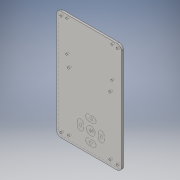
# Autodesk Inventor part: FrontCover
Saved by Autodesk Inventor 2016 (Build 200138000, 138)
## iProperties
Created: 2016-07-10
Part Number: FrontCover
Material: Generic
Document SubType Name: Modeling
Designer: jeffkub
Density: 1 g/cm^3
Appearance: Default
Author: jeffkub
Autodesk Inventor part; units mm, degrees
ref_plane "YZ Plane" through (0, 0, 0) normal (1, 0, 0) x (0, 1, 0)
ref_plane "XZ Plane" through (0, 0, 0) normal (0, 1, 0) x (-1, 0, 0)
ref_plane "XY Plane" through (0, 0, 0) normal (0, 0, 1) x (1, 0, 0)
sketch "Sketch1" plane through (0, 0, 0) normal (0, 0, 1) x (1, 0, 0)
  line L0 (30.48, -47.625) -> (-30.48, -47.625) construction
  line L1 (-34.925, -43.18) -> (-34.925, 43.18) construction
  line L2 (-30.48, 47.625) -> (30.48, 47.625) construction
  line L3 (34.925, 43.18) -> (34.925, -43.18) construction
  line L4 (34.925, -47.625) -> (-34.925, 47.625) construction
  line L5 (-34.925, -47.625) -> (34.925, 47.625) construction
  arc A0 (-30.48, 47.625) -> (-34.925, 43.18) centre (-30.48, 43.18) ccw construction
  arc A1 (34.925, 43.18) -> (30.48, 47.625) centre (30.48, 43.18) ccw construction
  arc A2 (30.48, -47.625) -> (34.925, -43.18) centre (30.48, -43.18) ccw construction
  arc A3 (-34.925, -43.18) -> (-30.48, -47.625) centre (-30.48, -43.18) ccw construction
  circle A4 centre (-30.48, 43.18) radius 1.5
  circle A5 centre (30.48, 43.18) radius 1.5
  circle A6 centre (-30.48, -43.18) radius 1.5
  circle A7 centre (30.48, -43.18) radius 1.5
  circle A8 centre (0, -22.86) radius 6.35
  line L6 (-3.175, -7.62) -> (3.175, -7.62) construction
  line L7 (-3.175, -12.065) -> (3.175, -12.065)
  line L8 (3.175, -3.175) -> (-3.175, -3.175)
  arc A9 (-3.175, -3.175) -> (-3.175, -12.065) centre (-3.175, -7.62) ccw
  arc A10 (3.175, -12.065) -> (3.175, -3.175) centre (3.175, -7.62) ccw
  line L9 (-35.3, 57.15) -> (35.3, 57.15) construction
  line L10 (35.3, 57.15) -> (35.3, 106.85) construction
  line L11 (35.3, 106.85) -> (-35.3, 106.85) construction
  line L12 (-35.3, 106.85) -> (-35.3, 57.15) construction
  circle A11 centre (-33.25, 104.75) radius 1.25
  circle A12 centre (33.25, 104.75) radius 1.25
  circle A13 centre (33.25, 59.25) radius 1.25
  circle A14 centre (-33.25, 59.25) radius 1.25
  line L13 (-41.275, 110.025) -> (41.275, 110.025)
  line L14 (47.625, 103.675) -> (47.625, -44.45)
  line L15 (41.275, -50.8) -> (-41.275, -50.8)
  line L16 (-47.625, -44.45) -> (-47.625, 103.675)
  arc A15 (-41.275, 110.025) -> (-47.625, 103.675) centre (-41.275, 103.675) ccw
  arc A16 (47.625, 103.675) -> (41.275, 110.025) centre (41.275, 103.675) ccw
  arc A17 (41.275, -50.8) -> (47.625, -44.45) centre (41.275, -44.45) ccw
  arc A18 (-47.625, -44.45) -> (-41.275, -50.8) centre (-41.275, -44.45) ccw
  circle A19 centre (-41.275, 103.675) radius 1.5
  circle A20 centre (-41.275, -44.45) radius 1.5
  circle A21 centre (41.275, -44.45) radius 1.5
  circle A22 centre (41.275, 103.675) radius 1.5
  line L17 (-0.635, -22.225) -> (-0.635, -20.32)
  line L18 (-0.635, -20.32) -> (-3.175, -22.86)
  line L19 (-3.175, -22.86) -> (-0.635, -25.4)
  line L20 (-0.635, -25.4) -> (-0.635, -23.495)
  line L21 (-0.635, -23.495) -> (3.175, -23.495)
  line L22 (3.175, -23.495) -> (3.175, -20.32)
  line L23 (3.175, -20.32) -> (1.905, -20.32)
  line L24 (1.905, -20.32) -> (1.905, -22.225)
  line L25 (1.905, -22.225) -> (-0.635, -22.225)
  line L26 (-2.54, -8.89) -> (2.54, -8.89)
  line L27 (2.54, -8.89) -> (2.54, -7.62)
  line L28 (2.54, -7.62) -> (0, -5.08)
  line L29 (0, -5.08) -> (-2.54, -7.62)
  line L30 (-2.54, -7.62) -> (-2.54, -8.89)
  arc A23 (-19.685, -26.035) -> (-10.795, -26.035) centre (-15.24, -26.035) ccw
  line L31 (-19.685, -19.685) -> (-19.685, -26.035)
  arc A24 (-10.795, -19.685) -> (-19.685, -19.685) centre (-15.24, -19.685) ccw
  line L32 (-10.795, -26.035) -> (-10.795, -19.685)
  line L33 (-13.97, -25.4) -> (-13.97, -20.32)
  line L34 (-13.97, -20.32) -> (-15.24, -20.32)
  line L35 (-15.24, -20.32) -> (-17.78, -22.86)
  line L36 (-17.78, -22.86) -> (-15.24, -25.4)
  line L37 (-15.24, -25.4) -> (-13.97, -25.4)
  arc A25 (3.175, -42.545) -> (3.175, -33.655) centre (3.175, -38.1) ccw
  line L38 (-3.175, -42.545) -> (3.175, -42.545)
  arc A26 (-3.175, -33.655) -> (-3.175, -42.545) centre (-3.175, -38.1) ccw
  line L39 (3.175, -33.655) -> (-3.175, -33.655)
  line L40 (2.54, -36.83) -> (-2.54, -36.83)
  line L41 (-2.54, -36.83) -> (-2.54, -38.1)
  line L42 (-2.54, -38.1) -> (0, -40.64)
  line L43 (0, -40.64) -> (2.54, -38.1)
  line L44 (2.54, -38.1) -> (2.54, -36.83)
  arc A27 (19.685, -19.685) -> (10.795, -19.685) centre (15.24, -19.685) ccw
  line L45 (19.685, -26.035) -> (19.685, -19.685)
  arc A28 (10.795, -26.035) -> (19.685, -26.035) centre (15.24, -26.035) ccw
  line L46 (10.795, -19.685) -> (10.795, -26.035)
  line L47 (13.97, -20.32) -> (13.97, -25.4)
  line L48 (13.97, -25.4) -> (15.24, -25.4)
  line L49 (15.24, -25.4) -> (17.78, -22.86)
  line L50 (17.78, -22.86) -> (15.24, -20.32)
  line L51 (15.24, -20.32) -> (13.97, -20.32)
  line L52 (5.205, 21.035) -> (16.385, 21.035) construction
  line L53 (16.385, 21.035) -> (16.385, 36.115) construction
  line L54 (16.385, 36.115) -> (5.205, 36.115) construction
  line L55 (5.205, 36.115) -> (5.205, 21.035) construction
  line L56 (5.205, 21.035) -> (16.385, 36.115) construction
  line L57 (16.385, 21.035) -> (5.205, 36.115) construction
  line L58 (20.265, 22.71) -> (29.265, 22.71) construction
  line L59 (29.265, 22.71) -> (29.265, 33.61) construction
  line L60 (29.265, 33.61) -> (20.265, 33.61) construction
  line L61 (20.265, 33.61) -> (20.265, 22.71) construction
  line L62 (-7.495, 36.115) -> (-7.495, 21.035) construction
  line L63 (3.685, 36.115) -> (-7.495, 36.115) construction
  line L64 (3.685, 21.035) -> (3.685, 36.115) construction
  line L65 (-7.495, 21.035) -> (3.685, 21.035) construction
  line L66 (-20.195, 36.115) -> (-20.195, 21.035) construction
  line L67 (-9.015, 36.115) -> (-20.195, 36.115) construction
  line L68 (-9.015, 21.035) -> (-9.015, 36.115) construction
  line L69 (-20.195, 21.035) -> (-9.015, 21.035) construction
  line L70 (-32.895, 36.115) -> (-32.895, 21.035) construction
  line L71 (-21.715, 36.115) -> (-32.895, 36.115) construction
  line L72 (-21.715, 21.035) -> (-21.715, 36.115) construction
  line L73 (-32.895, 21.035) -> (-21.715, 21.035) construction
  line L74 (-33.657, 37.385) -> (17.147, 37.385)
  line L75 (17.655, 36.877) -> (17.655, 35.388)
  line L76 (18.163, 34.88) -> (30.027, 34.88)
  line L77 (30.535, 34.372) -> (30.535, 21.948)
  line L78 (30.027, 21.44) -> (18.163, 21.44)
  line L79 (17.655, 20.932) -> (17.655, 20.273)
  line L80 (17.147, 19.765) -> (-33.657, 19.765)
  line L81 (-34.165, 20.273) -> (-34.165, 36.877)
  arc A29 (-33.657, 37.385) -> (-34.165, 36.877) centre (-33.657, 36.877) ccw
  arc A30 (17.655, 36.877) -> (17.147, 37.385) centre (17.147, 36.877) ccw
  arc A31 (17.655, 35.388) -> (18.163, 34.88) centre (18.163, 35.388) ccw
  arc A32 (30.535, 34.372) -> (30.027, 34.88) centre (30.027, 34.372) ccw
  arc A33 (30.027, 21.44) -> (30.535, 21.948) centre (30.027, 21.948) ccw
  arc A34 (18.163, 21.44) -> (17.655, 20.932) centre (18.163, 20.932) ccw
  arc A35 (17.147, 19.765) -> (17.655, 20.273) centre (17.147, 20.273) ccw
  arc A36 (-34.165, 20.273) -> (-33.657, 19.765) centre (-33.657, 20.273) ccw
  line L82 (-41.1, 50.8) -> (-38.1, 50.8)
  line L83 (-38.1, 50.8) -> (-38.1, 31.75)
  line L84 (-38.1, -38.1) -> (-41.1, -38.1)
  line L85 (-41.1, -38.1) -> (-41.1, -19.05)
  line L86 (-41.1, 31.75) -> (-38.1, 31.75)
  line L87 (-41.1, -19.05) -> (-38.1, -19.05)
  line L88 (-41.1, 31.75) -> (-41.1, 50.8)
  line L89 (-41.1, -19.05) -> (-41.1, 31.75) construction
  line L90 (-38.1, -19.05) -> (-38.1, -38.1)
  line L91 (-38.1, 31.75) -> (-38.1, -19.05) construction
  circle A37 centre (-39.6, 6.35) radius 1.5
  line L92 (0, -68.4111) -> (0, 116.4523)
  line L93 (41.1, 50.8) -> (38.1, 50.8)
  line L94 (38.1, 50.8) -> (38.1, 31.75)
  line L95 (38.1, -38.1) -> (41.1, -38.1)
  line L96 (41.1, -38.1) -> (41.1, -19.05)
  line L97 (41.1, 31.75) -> (38.1, 31.75)
  line L98 (41.1, -19.05) -> (38.1, -19.05)
  line L99 (41.1, 31.75) -> (41.1, 50.8)
  line L100 (38.1, -19.05) -> (38.1, -38.1)
  circle A38 centre (39.6, 6.35) radius 1.5
  point P0 (0, 0)
  point P1 (0, 0)
  point P2 (0, -7.62)
  point P3 (0, 57.15)
  point P4 (0, 0)
  point P5 (35.3, 82)
  point P6 (0, -8.89)
  point P7 (-13.97, -22.86)
  point P8 (0, -36.83)
  point P9 (13.97, -22.86)
  point P10 (10.795, 28.575)
  point P11 (24.765, 29.21)
  point P12 (24.765, 33.61)
  point P13 (-38.1, 6.35)
  point P14 (-39.6, 50.8)
  dimension "d0" = 69.85
  dimension "d1" = 95.25
  dimension "d2" = 4.445
  dimension "d3" = 3
  dimension "d4" = 24.765
  dimension "d5" = 12.7
  dimension "d6" = 6.35
  dimension "d7" = 8.89
  dimension "d8" = 15.24
  dimension "d9" = 70.6
  dimension "d10" = 49.7
  dimension "d11" = 9.525
  dimension "d12" = 66.5
  dimension "d13" = 33.25
  dimension "d14" = 45.5
  dimension "d15" = 22.75
  dimension "d16" = 2.5
  dimension "d17" = 3.175
  dimension "d18" = 12.7
  dimension "d19" = 3.175
  dimension "d20" = 12.7
  dimension "d21" = 6.35
  dimension "d22" = 3
  dimension "d25" = 1.27
  dimension "d26" = 1.27
  dimension "d27" = 0.635
  dimension "d28" = 0.635
  dimension "d29" = 5.08
  dimension "d30" = 2.54
  dimension "d31" = 3.81
  dimension "d32" = 3.175
  dimension "d33" = 5.08
  dimension "d34" = 1.27
  dimension "d35" = 2.54
  dimension "d38" = 360
  dimension "d42" = 11.18
  dimension "d43" = 15.08
  dimension "d44" = 19.05
  dimension "d45" = 24.13
  dimension "d54" = 6.5
  dimension "d55" = 10.9
  dimension "d56" = 9
  dimension "d57" = 10.16
  dimension "d58" = 18.415
  dimension "d61" = 12.7
  dimension "d66" = 1.27
  dimension "d67" = 1.27
  dimension "d68" = 1.27
  dimension "d69" = 1.27
  dimension "d70" = 1.27
  dimension "d71" = 1.27
  dimension "d72" = 1.27
  dimension "d73" = 0.508
  dimension "d74" = 3
  dimension "d76" = 12.7
  dimension "d77" = 88.9
  dimension "d78" = 19.05
  dimension "d79" = 19.05
  dimension "d80" = 3
  dimension "d81" = 76.2
  constraints: 204 end point, 48 point on circle, 39 centre point, 36 tangent, 28 perpendicular, 22 equal radius, 21 parallel, 13 midpoint, 13 point on line, 10 horizontal, 9 symmetric about line, 9 vertical alignment, 8 coincident, 4 horizontal alignment, 2 collinear, 2 vertical, 110 other
  measures "d0" distance of L4.end L5.end
  measures "d1" distance of L5.end L4.start
  measures "d2" radius of A0
  measures "d3" diameter of A4
  measures "d4" distance from line of L0 A8.centre
  measures "d5" diameter of A8
  measures "d6" distance of L6.start L6.end
  measures "d7" distance between parallel lines of L7 L8
  measures "d8" distance from line of A8.centre L6
  measures "d9" distance of L10.end L11.end
  measures "d10" distance of L9.end L10.end
  measures "d11" distance between parallel lines of L2 L9
  measures "d12" distance of A12.centre A11.centre
  measures "d13" horizontal distance of point (0, 57.15) A11.centre
  measures "d14" distance of A13.centre A12.centre
  measures "d15" vertical distance of point (35.3, 82) A12.centre
  measures "d16" diameter of A11
  measures "d17" distance between parallel lines of L13 L11
  measures "d18" distance between parallel lines of L14 L3
  measures "d19" distance between parallel lines of L15 L0
  measures "d20" distance between parallel lines of L16 L1
  measures "d21" radius of A15
  measures "d22" diameter of A19
  measures "d25" distance of L22.end L23.end
  measures "d26" distance between parallel lines of L21 L25
  measures "d27" distance from line of A8.centre L17
  measures "d28" distance from line of L25 A8.centre
  measures "d29" distance of L19.end L17.end
  measures "d30" distance from line of L17 L18.end
  measures "d31" distance of L20.end L21.end
  measures "d32" distance of L21.end L22.end
  measures "d33" distance of L26.start L26.end
  measures "d34" distance of L26.end L27.end
  measures "d35" horizontal distance of L27.end L28.end
  measures "d42" distance of L53.end L54.end
  measures "d43" distance of L52.end L53.end
  measures "d44" distance from line of point (10.795, 28.575) L2
  measures "d45" distance from line of L3 point (10.795, 28.575)
  measures "d54" distance from line of L58 point (24.765, 29.21)
  measures "d55" distance of L58.end L59.end
  measures "d56" distance of L59.end L60.end
  measures "d57" distance from line of L3 point (24.765, 29.21)
  measures "d58" distance from line of point (24.765, 29.21) L2
  measures "d61" distance of L54.end L62.start
  measures "d66" distance between parallel lines of L74 L71
  measures "d67" distance between parallel lines of L81 L70
  measures "d68" distance between parallel lines of L80 L73
  measures "d69" distance between parallel lines of L53 L79
  measures "d70" distance between parallel lines of L58 L78
  measures "d71" distance between parallel lines of L77 L59
  measures "d72" distance between parallel lines of L76 L60
  measures "d73" radius of A29
  measures "d74" distance of L82.start L82.end
  measures "d76" distance between parallel lines of L84 L15
  measures "d77" distance between parallel lines of L84 L82
  measures "d78" distance between parallel lines of L84 L87
  measures "d79" distance between parallel lines of L86 L82
  measures "d80" diameter of A37
  measures "d81" diameter of L90 L92
extrude "Extrusion1" add sketch "Sketch1" along normal blind 3 contours A8 L92 L21 L22 L23 L24 L25 | A8 L92 L7 A10 L8 L80 A35 L79 A34 L78 A33 L77 A32 L76 A31 L75 A30 L74 L13 A16 L14 A17 L15 L38 A25 L39 | L92 L25 L17 L18 L19 L20 L21 A8 | A8 L92 L39 A26 L38 L15 A18 L16 A15 L13 L74 A29 L81 A36 L80 L8 A9 L7 | L92 L21 L20 L19 L18 L17 L25 | L25 L24 L23 L22 L21 L92 | L92 L26 L27 L28 L8 A10 L7 | L7 A9 L8 L92 L29 L30 L26 | L92 L40 L41 L42 L38 A26 L39 | L39 A25 L38 L92 L43 L44 L40 | L92 L28 L27 L26 | L26 L30 L29 L92 | L92 L42 L41 L40 | L40 L44 L43 L92 | L92 L74 A30 L75 A31 L76 A32 L77 A33 L78 A34 L79 A35 L80 | L80 A36 L81 A29 L74 L92 | L31 A24 L32 A23 | L37 L36 L35 L34 L33 | L45 A28 L46 A27 | L51 L50 L49 L48 L47 | L82 L83 L86 L88 | L84 L85 L87 L90 | A37 | L99 L97 L94 L93 | L100 L98 L96 L95 | A38
extrude "Extrusion2" cut sketch "Sketch1" along normal blind 0.5 contours A8 L92 L21 L22 L23 L24 L25 | L92 L25 L17 L18 L19 L20 L21 A8 | L92 L26 L27 L28 L8 A10 L7 | L7 A9 L8 L92 L29 L30 L26 | L92 L40 L41 L42 L38 A26 L39 | L39 A25 L38 L92 L43 L44 L40 | L31 A24 L32 A23 | L45 A28 L46 A27
sketch "Sketch2" plane through (0, 0, 3) normal (0, 0, 1) x (1, 0, 0)
  circle A0 centre (41.275, 103.675) radius 1.5 projected
  circle A1 centre (41.275, -44.45) radius 1.5 projected
  circle A2 centre (-41.275, -44.45) radius 1.5 projected
  circle A3 centre (-41.275, 103.675) radius 1.5 projected
  circle A4 centre (30.48, -43.18) radius 1.5 projected
  circle A5 centre (-30.48, -43.18) radius 1.5 projected
  circle A6 centre (30.48, 43.18) radius 1.5 projected
  circle A7 centre (-30.48, 43.18) radius 1.5 projected
  circle A8 centre (-33.25, 59.25) radius 1.25 projected
  circle A9 centre (33.25, 59.25) radius 1.25 projected
  circle A10 centre (33.25, 104.75) radius 1.25 projected
  circle A11 centre (-33.25, 104.75) radius 1.25 projected
  line L0 (41.275, 110.025) -> (-41.275, 110.025) projected
  arc A12 (-41.275, 110.025) -> (-47.625, 103.675) centre (-41.275, 103.675) ccw projected
  line L1 (-47.625, 103.675) -> (-47.625, -44.45) projected
  arc A13 (-47.625, -44.45) -> (-41.275, -50.8) centre (-41.275, -44.45) ccw projected
  line L2 (-41.275, -50.8) -> (41.275, -50.8) projected
  arc A14 (41.275, -50.8) -> (47.625, -44.45) centre (41.275, -44.45) ccw projected
  line L3 (47.625, -44.45) -> (47.625, 103.675) projected
  arc A15 (47.625, 103.675) -> (41.275, 110.025) centre (41.275, 103.675) ccw projected
  line L4 (-41.275, 110.125) -> (41.275, 110.125)
  arc A16 (47.725, 103.675) -> (41.275, 110.125) centre (41.275, 103.675) ccw
  line L5 (47.725, 103.675) -> (47.725, -44.45)
  arc A17 (41.275, -50.9) -> (47.725, -44.45) centre (41.275, -44.45) ccw
  line L6 (41.275, -50.9) -> (-41.275, -50.9)
  arc A18 (-47.725, -44.45) -> (-41.275, -50.9) centre (-41.275, -44.45) ccw
  line L7 (-47.725, -44.45) -> (-47.725, 103.675)
  arc A19 (-41.275, 110.125) -> (-47.725, 103.675) centre (-41.275, 103.675) ccw
  point P0 (0, 0)
  dimension "d82" = 0.1
  constraints: 8 end point, 8 point on circle, 4 centre point, 7 other
  measures "d82" distance between parallel lines of L0 L4
extrude "Extrusion3" add sketch "Sketch2" against normal up to surface (3 mm away) contours L4 A16 L5 A17 L6 A18 L7 A19
equation "\"d13\" = 0.5 * d12"
equation "\"d15\" = 0.5 * d14"
equation "\"d19\" = d17"
equation "\"d20\" = d18"
equation "\"d28\" = 0.5 * d26"
equation "\"d67\" = d66"
equation "\"d68\" = d66"
equation "\"d69\" = d66"
equation "\"d70\" = d66"
equation "\"d71\" = d66"
equation "\"d72\" = d66"
equation "\"d78\" = d79"
body "Solid1"
